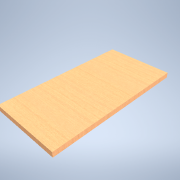
# Autodesk Inventor part: Creat Buttom
Saved by Autodesk Inventor 2021 (Build 250183000, 183)
## iProperties
Created: 2020-08-15
Part Number: Creat Buttom
Material: Wood (Cherry)
Document SubType Name: Modeling
Designer: Oghenemarho
Density: 0.63 g/cm^3
Appearance: Cherry - Natural Low Gloss
Author: Oghenemarho
Autodesk Inventor part; units mm, degrees
ref_plane "YZ Plane" through (0, 0, 0) normal (1, 0, 0) x (0, 1, 0)
ref_plane "XZ Plane" through (0, 0, 0) normal (0, 1, 0) x (-1, 0, 0)
ref_plane "XY Plane" through (0, 0, 0) normal (0, 0, 1) x (1, 0, 0)
sketch "Sketch1" plane through (0, 0, 0) normal (0, 1, 0) x (-1, 0, 0)
  line L0 (-125, 250) -> (125, 250)
  line L1 (125, 250) -> (125, -250)
  line L2 (125, -250) -> (-125, -250)
  line L3 (-125, -250) -> (-125, 250)
  line L4 (-125, 250) -> (125, -250) construction
  line L5 (125, 250) -> (-125, -250) construction
  point P0 (0, 0)
  dimension "Width" = 250
  dimension "lenght" = 500
  constraints: 12 end point, 2 midpoint, 2 parallel, 1 horizontal, 1 perpendicular
  measures "Width" distance of L1.end L2.end
  measures "lenght" distance of L2.end L0.start
extrude "Extrusion1" add sketch "Sketch1" along normal blind 19.05
body "Solid1"
